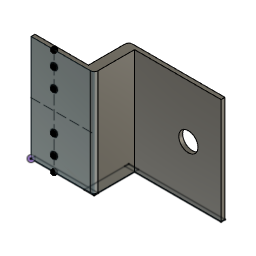
drox-tail v1 (Autodesk Fusion 360 design; units mm, degrees)
Autodesk Fusion 360 part; units mm, degrees
sketch "Sketch1" plane through (0, 0, 0) normal (0, 0, 1) x (1, 0, 0)
  line L0 (0, 0) -> (32.8, 0)
  line L1 (32.8, 0) -> (32.8, 2)
  line L2 (32.8, 2) -> (0, 2)
  line L3 (0, 2) -> (0, 0)
  line L4 (32.8, 0) -> (27.8, 0)
  line L5 (27.8, 0) -> (27.8, 23)
  line L6 (27.8, 23) -> (32.8, 23)
  line L7 (32.8, 23) -> (32.8, 0)
  line L8 (27.8, 23) -> (77.8, 23)
  line L9 (77.8, 23) -> (77.8, 21)
  line L10 (77.8, 21) -> (27.8, 21)
  line L11 (27.8, 21) -> (27.8, 23)
  dimension "d1" = 32.8
  dimension "d2" = 2
  dimension "d3" = 5
  dimension "d4" = 23
  dimension "d5" = 50
  dimension "d6" = 2
  constraint horizontal L0
  constraint vertical L1
  constraint horizontal L2
  constraint vertical L3
  constraint coincident L0.start L3.end
  constraint horizontal L4
  constraint vertical L5
  constraint horizontal L6
  constraint vertical L7
  constraint horizontal L8
  constraint vertical L9
  constraint horizontal L10
  constraint vertical L11
  measures "d1" distance of L0.start L0.end
  measures "d2" distance of L0.start L2.end
  measures "d3" distance of L0.end L4.end
  measures "d4" distance of L0.end L6.end
  measures "d5" distance of L5.end L8.end
  measures "d6" distance of L5.end L10.end
extrude "Extrude1" add sketch "Sketch1" along normal blind 55
sketch "Sketch2" plane through (0, 0, 0) normal (0, -1, 0) x (1, 0, 0)
  line L0 (0, 0) -> (32.8, 0)
  line L1 (32.8, 0) -> (32.8, 55)
  line L2 (32.8, 55) -> (0, 55)
  line L3 (0, 55) -> (0, 0)
  line L4 (12, 55) -> (12, 0) construction
  line L5 (0, 27.5) -> (32.8, 27.5) construction
  circle A0 centre (12, 47.5) radius 1.6
  circle A1 centre (12, 37.5) radius 1.6
  circle A2 centre (12, 17.5) radius 1.6
  circle A3 centre (12, 7.5) radius 1.6
  dimension "d10" = 3.2
  dimension "d11" = 3.2
  dimension "d12" = 3.2
  dimension "d13" = 3.2
  dimension "d14" = 10
  dimension "d15" = 10
  dimension "d17" = 10
  dimension "d19" = 10
  dimension "d30" = 12
  constraint coincident L2 L4.start
  constraint perpendicular L2 L4
  constraint coincident L0 L4.end
  constraint midpoint L3 L5.start
  constraint midpoint L1 L5.end
  constraint coincident L4 A0.centre
  constraint coincident L4 A1.centre
  constraint coincident L4 A2.centre
  constraint coincident L4 A3.centre
  measures "d10" diameter of A0
  measures "d11" diameter of A1
  measures "d12" diameter of A2
  measures "d13" diameter of A3
  measures "d14" distance of L5 A1.centre
  measures "d15" distance of A0.centre A1.centre
  measures "d17" distance of L5 A2.centre
  measures "d19" distance of A2.centre A3.centre
  measures "d30" distance of L3 L4
extrude "Extrude2" cut sketch "Sketch2" against normal blind 25 contours A0 | A1 | A2 | A3
fillet "Fillet1" radius 2 1 edges at (32.8, 0, 27.5)
fillet "Fillet2" radius 2 1 edges at (27.8, 23, 27.5)
sketch "Sketch3" plane through (0, 21, 0) normal (0, -1, 0) x (1, 0, 0)
  line L0 (32.8, 0) -> (77.8, 0)
  line L1 (77.8, 0) -> (77.8, 55)
  line L2 (77.8, 55) -> (32.8, 55)
  line L3 (32.8, 55) -> (32.8, 0)
  line L4 (60.8, 55) -> (60.8, 0) construction
  line L5 (77.8, 27.5) -> (32.8, 27.5) construction
  circle A0 centre (60.8, 27.5) radius 5
  dimension "d26" = 28
  dimension "d27" = 10
  constraint coincident L2 L4.start
  constraint perpendicular L2 L4
  constraint coincident L0 L4.end
  constraint midpoint L1 L5.start
  constraint midpoint L3 L5.end
  constraint midpoint L4 A0.centre
  measures "d26" distance of L3 L4
  measures "d27" diameter of A0
extrude "Extrude3" cut sketch "Sketch3" against normal blind 15 contours A0
equation "bodyScrew = 3.2 mm"
equation "d10 = bodyScrew"
equation "d11 = bodyScrew"
equation "d12 = bodyScrew"
equation "d13 = bodyScrew"
